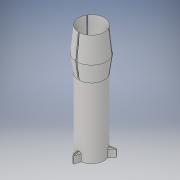
# Autodesk Inventor part: Engine_Holder_Mk_II
Saved by Autodesk Inventor 2017 (Build 210142000, 142)
## iProperties
Created: 2017-04-26
Part Number: Engine_Holder_Mk_II
Material: Generic
Document SubType Name: Modeling
Designer: seane
Density: 1 g/cm^3
Appearance: Default
Author: seane
Autodesk Inventor part; units mm, degrees
ref_plane "YZ Plane" through (0, 0, 0) normal (1, 0, 0) x (0, 1, 0)
ref_plane "XZ Plane" through (0, 0, 0) normal (0, 1, 0) x (-1, 0, 0)
ref_plane "XY Plane" through (0, 0, 0) normal (0, 0, 1) x (1, 0, 0)
sketch "Sketch1" plane through (0, 0, 0) normal (1, 0, 0) x (0, 1, 0)
  line L0 (0, 0) -> (0, -12.065)
  line L1 (0, -12.065) -> (91.44, -12.065)
  line L2 (91.44, -12.065) -> (91.44, -13.335)
  line L3 (91.44, -13.335) -> (0, -13.335)
  line L4 (0, -13.335) -> (0, -12.065)
  line L5 (0, 0) -> (110.5631, 0)
  line L6 (91.44, -13.335) -> (116.84, -13.335)
  line L7 (91.44, -13.335) -> (91.44, -15.875)
  line L8 (91.44, -15.875) -> (116.84, -13.335)
  line L9 (91.44, -15.875) -> (73.3806, -13.335)
  dimension "d0" = 12.065
  dimension "d1" = 91.44
  dimension "d2" = 1.27
  dimension "d3" = 25.4
  dimension "d4" = 2.54
  constraints: 20 end point, 4 perpendicular, 2 horizontal, 2 point on line, 2 vertical
  measures "d0" distance of L0.start L0.end
  measures "d1" distance of L0.end L1.end
  measures "d2" distance of L1.end L2.end
  measures "d3" distance of L2.end L6.end
  measures "d4" distance of L2.end L7.end
revolve "Revolution1" add sketch "Sketch1" angle 360 about axis through (0, 0, 0) along (0, 1, 0)
sketch "Sketch2" plane through (0, 0, 0) normal (0, -1, 0) x (1, 0, 0)
  circle A0 centre (0, 0) radius 13.335
  line L0 (11.2178, -7.2099) -> (16.1473, -10.0559)
  line L1 (11.8528, -6.11) -> (16.7823, -8.9561)
  line L2 (0.635, 13.3199) -> (0.635, 19.012)
  line L3 (-0.635, 13.3199) -> (-0.635, 19.012)
  line L4 (-11.8528, -6.11) -> (-16.7823, -8.9561)
  line L5 (-11.2178, -7.2099) -> (-16.1473, -10.0559)
  line L6 (16.1473, -10.0559) -> (16.7823, -8.9561)
  line L7 (0.635, 19.012) -> (-0.635, 19.012)
  line L8 (-16.7823, -8.9561) -> (-16.1473, -10.0559)
  line L9 (-0.635, 19.012) -> (-2.2892, 13.137)
  circle A1 centre (0, 0) radius 13.335 projected
  line L10 (0.635, 19.012) -> (2.2723, 13.14)
  line L11 (16.7823, -8.9561) -> (12.5157, -4.6021)
  line L12 (-16.1473, -10.0559) -> (-10.2434, -8.5379)
  line L13 (-16.7823, -8.9561) -> (-12.5157, -4.6021)
  line L14 (16.1473, -10.0559) -> (10.2434, -8.5379)
  dimension "d24" = 6.096
  dimension "d25" = 6.096
  dimension "d27" = 6.096
  dimension "d28" = 6.096
  dimension "d29" = 6.096
  constraints: 30 end point, 6 point on circle, 1 coincident, 1 horizontal, 9 other
  measures "d24" distance of L2.end L10.end
  measures "d25" distance of L1.end L11.end
  measures "d27" distance of L5.end L12.end
  measures "d28" distance of L4.end L13.end
  measures "d29" distance of L0.end L14.end
extrude "Extrusion1" add sketch "Sketch2" against normal blind 8.89 contours A0 L2 L10 | L11 L1 A0 | A0 L9 L3 | L0 L14 A0 | A0 L4 L13 | L12 L5 A0
extrude "Extrusion2" cut sketch "Sketch2" against normal blind 124.7775 contours A0 L3 L7 L2 | L1 L6 L0 A0 | A0 L5 L8 L4
chamfer "Chamfer1" distance 1.397 angle 45 6 edges at (1.4537, 8.89, 16.076) (-1.4621, 8.89, 16.0745) (14.649, 8.89, -6.7791) (13.1954, 8.89, -9.2969) (-13.1954, 8.89, -9.2969) (-14.649, 8.89, -6.7791)
body "Solid1"
